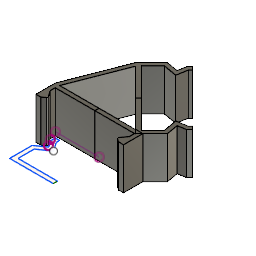
wireductbracket (Autodesk Fusion 360 design; units mm, degrees)
Autodesk Fusion 360 part; units mm, degrees
note: some values were not read from the file. Set by a fixed rule: which sketch regions a step uses.
sketch "Sketch1" plane through (0, 0, 0) normal (0, 0, 1) x (1, 0, 0)
  line L0 (-9.5, 2.7412) -> (-9.5, 1.5138)
  line L1 (-9.5, 1.5138) -> (-8.4721, 0.0457)
  line L2 (-8.5457, -0.3721) -> (-9.2969, -0.8981)
  line L3 (-9.5, 2.7412) -> (0.0002, 2.7412)
  line L4 (-9.2969, -0.8981) -> (-10.5, -0.8981)
  line L5 (-10.5, -0.8981) -> (-10.5, 3.7412)
  line L6 (-10.5, 3.7412) -> (0.0002, 3.7412)
  line L7 (0.0002, 3.7412) -> (0.0002, 2.7412)
  arc A0 (-8.5457, -0.3721) -> (-8.4721, 0.0457) centre (-8.7178, -0.1263) ccw
  point P0 (-8.3, -0.2)
  dimension "d1" = 145
  dimension "d2" = 1
  dimension "d3" = 1
  dimension "d7" = 8.3
  dimension "d8" = 10.5
  dimension "d33" = 145
  dimension "d34" = 0.3
  measures "d1" angle of L0 L1
  measures "d2" distance of L3 L6
  measures "d3" distance of L0 L5
  measures "d7" distance of origin P0
  measures "d8" distance of origin L5
  measures "d33" angle of L2 L4
  measures "d34" radius of A0
extrude "Extrude1" add sketch "Sketch1" along normal blind 10 makes body 1 in component "Component"
mirror "Mirror1" about plane through (0, 0, 0) normal (1, 0, 0) of bodies 1 makes body 2 in component "Component"
sketch "Sketch2" plane through (0, 0, 0) normal (0, 0, 1) x (1, 0, 0)
  line L0 (0.0002, 3.7412) -> (-10.5, 3.7412)
  line L1 (-9.2, 2.4161) -> (-9.2, 1.3343)
  line L2 (-8.4721, 0.0457) -> (-9.5, 1.5138)
  line L3 (-9.2, 1.3343) -> (-8.1019, -0.2339)
  line L4 (-8.1019, -0.2339) -> (-10.4422, -1.8726)
  line L5 (-10.4422, -1.8726) -> (-10.4422, -7.2624)
  line L6 (-10.4422, -7.2624) -> (0, -7.2624)
  line L7 (0, -7.2624) -> (0, -6.2624)
  line L8 (0, -6.2624) -> (-9.4422, -6.2624)
  line L9 (-9.4422, -6.2624) -> (-9.4422, -2.3931)
  line L10 (-9.4422, -2.3931) -> (-6.7065, -0.4776)
  line L11 (-6.7085, -0.4805) -> (-8.2, 1.6496)
  line L12 (-8.2, 1.6496) -> (-8.2, 2.4161)
  line L13 (-8.2, 2.4161) -> (-9.2, 2.4161)
  dimension "d13" = 1
  dimension "d14" = 1
  dimension "d19" = 125
  dimension "d20" = 1
  dimension "d21" = 1
  dimension "d22" = 1
  measures "d13" distance of L5 L9
  measures "d14" distance of L6 L8
  measures "d19" angle of L4 L5
  measures "d20" distance of L3 L11
  measures "d21" distance of L1 L12
  measures "d22" distance of L4 L10
extrude "Extrude2" add sketch "Sketch2" along normal blind 10 separate body makes body 3 in component "Component"
mirror "Mirror2" about plane through (0, 0, 0) normal (1, 0, 0) of bodies 3 makes body 4 in component "Component"
move_body "Move1" bodies 4 3 to x (0.707107, -0.707107, 0) y (0.707107, 0.707107, 0) z (0, 0, 1) at (7.3964, 15.368, 0) in component "Component"
sketch "Sketch3" plane through (0, 0, 0) normal (0, 0, 1) x (1, 0, 0)
  line L0 (-5.2632, 17.7165) -> (-10.6406, 3.8412)
  line L1 (-0.1404, 3.8412) -> (-10.6406, 3.8412)
  line L2 (-10.6406, 3.8412) -> (-9.5681, 3.8412)
  line L3 (-5.2632, 17.7165) -> (2.1205, 10.3327)
  line L4 (-4.4903, 16.9435) -> (-9.5681, 3.8412)
  point P0 (-5.2632, 17.7165)
  point P1 (-10.6406, 3.8412)
  dimension "d29" = 1
  measures "d29" distance of L0 L4
extrude "Extrude3" add sketch "Sketch3" along normal blind 10 sketch seen with x (1, 0, 0) y (0, 1, 0) z (0, 0, 1) at (0.1406, -0.1, 0) bodies 1 3 in component "Component"
component "Component" placed x (1, 0, 0) y (0, 1, 0) z (0, 0, 1) at (-0.1406, 0.1, 0)
equation "d8 = ( 21 / 2 ) * 1 mm"
